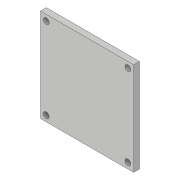
# Autodesk Inventor part: BASE FOR STORAGE SYSTEM
Saved by Autodesk Inventor 2019 (Build 230136000, 136)
## iProperties
Created: 2019-10-14
Part Number: BASE FOR STORAGE SYSTEM
Material: Generic
Document SubType Name: Modeling
Designer: Admin
Density: 1 g/cm^3
Appearance: Default
Author: Admin
Autodesk Inventor part; units mm, degrees
ref_plane "YZ Plane" through (0, 0, 0) normal (1, 0, 0) x (0, 1, 0)
ref_plane "XZ Plane" through (0, 0, 0) normal (0, 1, 0) x (-1, 0, 0)
ref_plane "XY Plane" through (0, 0, 0) normal (0, 0, 1) x (1, 0, 0)
sketch "Sketch1" plane through (0, 0, 0) normal (0, 0, 1) x (1, 0, 0)
  line L0 (0, 0) -> (160, 0)
  line L1 (160, 0) -> (160, 160)
  line L2 (160, 160) -> (0, 160)
  line L3 (0, 160) -> (0, 0)
  dimension "d0" = 160
  dimension "d1" = 160
  constraints: 8 end point, 2 parallel, 1 horizontal, 1 perpendicular
  measures "d0" distance of L2.end L1.end
  measures "d1" distance of L1.end L0.end
extrude "Extrusion1" add sketch "Sketch1" along normal blind 10
sketch "Sketch2" plane through (0, 0, 10) normal (0, 0, 1) x (1, 0, 0)
  line L0 (0, 0) -> (10, 0)
  line L1 (0, 0) -> (160, 0) projected
  line L2 (10, 0) -> (10, 10)
  line L3 (10, 10) -> (10, 150)
  line L4 (10, 150) -> (150, 150)
  line L5 (150, 150) -> (150, 10)
  line L6 (150, 10) -> (10, 10)
  circle A0 centre (10, 150) radius 5
  circle A1 centre (150, 150) radius 5
  circle A2 centre (150, 10) radius 5
  circle A3 centre (10, 10) radius 5
  dimension "d4" = 10
  dimension "d5" = 10
  dimension "d6" = 140
  dimension "d7" = 140
  dimension "d8" = 140
  dimension "d9" = 140
  dimension "d10" = 10
  dimension "d11" = 10
  dimension "d12" = 10
  dimension "d13" = 10
  constraints: 12 end point, 4 centre point, 4 coincident, 3 perpendicular, 2 point on line
  measures "d4" distance of L0.start L0.end
  measures "d5" distance of L0.end L2.end
  measures "d6" distance of L2.end L3.end
  measures "d7" distance of L3.end L4.end
  measures "d8" distance of L4.end L5.end
  measures "d9" distance of L5.end L2.end
  measures "d10" diameter of A0
  measures "d11" diameter of A1
  measures "d12" diameter of A2
  measures "d13" diameter of A3
extrude "Extrusion2" cut sketch "Sketch2" along normal through all both and the other way through all contours A3 L3 L2 | L2 L6 A3 | L3 A3 L6 | A0 L4 L3 | L3 L4 A0 | A2 L5 L6 | L6 L5 A2 | A1 L5 L4 | L4 L5 A1
body "Solid1"
